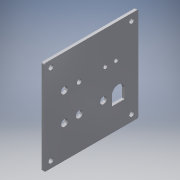
# Autodesk Inventor part: PP-LAS-0001
Saved by Autodesk Inventor 2018.3 (Build 223284000, 284)
## iProperties
Created: 2021-05-05
Part Number: PP-LAS-0001
Material: Plástico ABS
Document SubType Name: Modeling
Designer: L.Aguerre
Density: 1.06 g/cm^3
Appearance: Suave - Blanco
Description: FRENTE DE PANEL SERIGRAFIADO
Author: laguerre
Autodesk Inventor part; units mm, degrees
ref_plane "YZ Plane" through (0, 0, 0) normal (1, 0, 0) x (0, 1, 0)
ref_plane "XZ Plane" through (0, 0, 0) normal (0, 1, 0) x (-1, 0, 0)
ref_plane "XY Plane" through (0, 0, 0) normal (0, 0, 1) x (1, 0, 0)
sketch "Boceto39" plane through (0, 0, 0) normal (0, 0, 1) x (1, 0, 0)
  line L0 (-34, 35) -> (34, 35)
  line L1 (35, 34) -> (35, -34)
  line L2 (34, -35) -> (-34, -35)
  line L3 (-35, -34) -> (-35, 34)
  arc A0 (-34, 35) -> (-35, 34) centre (-34, 34) ccw
  arc A1 (35, 34) -> (34, 35) centre (34, 34) ccw
  arc A2 (34, -35) -> (35, -34) centre (34, -34) ccw
  arc A3 (-35, -34) -> (-34, -35) centre (-34, -34) ccw
  point P0 (0, 0)
  point P1 (0, 35)
  point P2 (-35, 0)
  dimension "d373" = 70
  dimension "d374" = 70
  dimension "d375" = 1
  constraints: 8 end point, 8 point on circle, 8 tangent, 4 centre point, 3 equal radius, 2 midpoint, 2 parallel, 1 horizontal, 1 horizontal alignment, 1 perpendicular, 1 vertical alignment
  measures "d373" distance between parallel lines of L1 L3
  measures "d374" distance between parallel lines of L2 L0
  measures "d375" radius of A0
extrude "Extrusión13" add sketch "Boceto39" along normal blind 2
sketch "Boceto43" plane through (0, 0, 2) normal (0, 0, 1) x (1, 0, 0)
  line L0 (-30, 30) -> (30, 30) construction
  line L1 (30, 30) -> (30, -30) construction
  line L2 (30, -30) -> (-30, -30) construction
  line L3 (-30, -30) -> (-30, 30) construction
  point P0 (0, 0)
  point P1 (0, 30)
  point P2 (-30, 0)
  dimension "d402" = 60
  constraints: 8 end point, 2 coincident, 2 midpoint, 2 parallel, 2 perpendicular, 1 horizontal, 1 horizontal alignment, 1 point on line, 1 vertical alignment
  measures "d402" distance of L0.start L0.end
hole "Agujero2" at (30, 30, 2) at (30, -30, 2) at (-30, -30, 2) at (-30, 30, 2) direction (0, 0, -1) diameter 3.5 depth 8 tip angle 118
sketch "Boceto40" plane through (0, 0, 2) normal (0, 0, 1) x (1, 0, 0)
  line L0 (-25, 0) -> (-4, 0)
  line L1 (-2, -2) -> (-2, -18)
  line L2 (-4, -20) -> (-25, -20)
  line L3 (-27, -18) -> (-27, -2)
  line L4 (4, 0) -> (25, 0)
  line L5 (27, -2) -> (27, -18)
  line L6 (25, -20) -> (4, -20)
  line L7 (2, -18) -> (2, -2)
  line L8 (-25, 20) -> (25, 20)
  line L9 (27, 18) -> (27, 5)
  line L10 (25, 3) -> (-25, 3)
  line L11 (-27, 5) -> (-27, 18)
  arc A0 (-27, -18) -> (-25, -20) centre (-25, -18) ccw
  arc A1 (-4, -20) -> (-2, -18) centre (-4, -18) ccw
  arc A2 (-2, -2) -> (-4, 0) centre (-4, -2) ccw
  arc A3 (-25, 0) -> (-27, -2) centre (-25, -2) ccw
  arc A4 (4, 0) -> (2, -2) centre (4, -2) ccw
  arc A5 (2, -18) -> (4, -20) centre (4, -18) ccw
  arc A6 (25, -20) -> (27, -18) centre (25, -18) ccw
  arc A7 (27, -2) -> (25, 0) centre (25, -2) ccw
  line L12 (-34, -35) -> (34, -35) projected
  arc A8 (-27, 5) -> (-25, 3) centre (-25, 5) ccw
  arc A9 (-25, 20) -> (-27, 18) centre (-25, 18) ccw
  arc A10 (27, 18) -> (25, 20) centre (25, 18) ccw
  arc A11 (25, 3) -> (27, 5) centre (25, 5) ccw
  line L13 (25, 19.7) -> (-25, 19.7)
  arc A12 (-25, 19.7) -> (-26.7, 18) centre (-25, 18) ccw
  line L14 (-26.7, 18) -> (-26.7, 5)
  arc A13 (-26.7, 5) -> (-25, 3.3) centre (-25, 5) ccw
  line L15 (-25, 3.3) -> (25, 3.3)
  arc A14 (25, 3.3) -> (26.7, 5) centre (25, 5) ccw
  line L16 (26.7, 5) -> (26.7, 18)
  arc A15 (26.7, 18) -> (25, 19.7) centre (25, 18) ccw
  line L17 (-4, -0.3) -> (-25, -0.3)
  arc A16 (-25, -0.3) -> (-26.7, -2) centre (-25, -2) ccw
  line L18 (-26.7, -2) -> (-26.7, -18)
  arc A17 (-26.7, -18) -> (-25, -19.7) centre (-25, -18) ccw
  line L19 (-25, -19.7) -> (-4, -19.7)
  arc A18 (-4, -19.7) -> (-2.3, -18) centre (-4, -18) ccw
  line L20 (-2.3, -18) -> (-2.3, -2)
  arc A19 (-2.3, -2) -> (-4, -0.3) centre (-4, -2) ccw
  line L21 (25, -0.3) -> (4, -0.3)
  arc A20 (4, -0.3) -> (2.3, -2) centre (4, -2) ccw
  line L22 (2.3, -2) -> (2.3, -18)
  arc A21 (2.3, -18) -> (4, -19.7) centre (4, -18) ccw
  line L23 (4, -19.7) -> (25, -19.7)
  arc A22 (25, -19.7) -> (26.7, -18) centre (25, -18) ccw
  line L24 (26.7, -18) -> (26.7, -2)
  arc A23 (26.7, -2) -> (25, -0.3) centre (25, -2) ccw
  point P0 (0, 0)
  point P1 (-27, 0)
  point P2 (-2, -20)
  point P3 (-27, -20)
  point P4 (27, -20)
  point P5 (2, -20)
  point P6 (0, 20)
  dimension "d378" = 2
  dimension "d379" = 2
  dimension "d380" = 25
  dimension "d381" = 25
  dimension "d382" = 20
  dimension "d383" = 2
  dimension "d385" = 3
  dimension "d386" = 2
  dimension "d387" = 17
  dimension "d388" = 0.3
  dimension "d389" = 0.3
  dimension "d390" = 0.3
  dimension "d477" = 20
  constraints: 48 end point, 48 point on circle, 24 centre point, 24 tangent, 12 parallel, 10 equal radius, 10 point on line, 6 perpendicular, 3 collinear, 3 horizontal, 1 midpoint, 1 vertical alignment, 21 other
  measures "d378" distance from line of point (0, 0) L1
  measures "d379" distance from line of point (0, 0) L7
  measures "d380" distance of point (-2, -20) point (-27, -20)
  measures "d381" distance of point (27, -20) point (2, -20)
  measures "d382" distance of point (-27, -20) point (-27, 0)
  measures "d383" radius of A0
  measures "d385" distance between parallel lines of L10 L0
  measures "d386" radius of A8
  measures "d387" distance between parallel lines of L8 L10
  measures "d388" distance between parallel lines of L15 L10
  measures "d389" distance between parallel lines of L4 L21
  measures "d390" distance between parallel lines of L0 L17
  measures "d477" distance from line of L6 point (0, 0)
extrude "Extrusión14" add sketch "Boceto40" along normal blind 0.001
sketch "Boceto41" plane through (0, 0, 2) normal (0, 0, 1) x (1, 0, 0)
  circle A0 centre (-20, -10.7) radius 5 construction
  line L0 (-34, -35) -> (34, -35) projected
  line L1 (-35, 34) -> (-35, -34) projected
  circle A1 centre (-9, -10.7) radius 2.5
  line L2 (-20, -10.7) -> (-9, -10.7) construction
  line L3 (-4, -19.7) -> (-25, -19.7) projected
  circle A2 centre (9, -10.7) radius 2.5
  circle A3 centre (20, -10.7) radius 2.5
  line L4 (25, -19.7) -> (4, -19.7) projected
  circle A4 centre (-18.5, 10.3) radius 1.5
  circle A5 centre (-10.5, 10.3) radius 1.5
  line L5 (-18.5, 10.3) -> (-10.5, 10.3) construction
  line L6 (25, 3.3) -> (-25, 3.3) projected
  circle A6 centre (20, 10.3) radius 2.5
  circle A7 centre (9, 10.3) radius 1.75
  line L7 (9, -10.7) -> (20, -10.7) construction
  line L8 (9, 10.3) -> (20, 10.3) construction
  line L9 (-24.7, -10.7) -> (-24.7, -17.7)
  line L10 (-24.7, -17.7) -> (-15.3, -17.7)
  line L11 (-15.3, -17.7) -> (-15.3, -10.7)
  arc A8 (-15.3, -10.7) -> (-24.7, -10.7) centre (-20, -10.7) ccw
  line L12 (-20, -6) -> (-22.9713, -6) construction
  point P0 (0, 0)
  point P1 (-14.5, -10.7)
  point P2 (-14.5, -19.7)
  point P3 (-14.5, 10.3)
  point P4 (14.5, -10.7)
  point P5 (14.5, -19.7)
  point P6 (14.5, 10.3)
  point P7 (-20, -17.7)
  dimension "d393" = 10
  dimension "d396" = 5
  dimension "d397" = 11
  dimension "d399" = 11
  dimension "d410" = 9
  dimension "d415" = 3
  dimension "d416" = 7
  dimension "d417" = 8
  dimension "d418" = 3.5
  dimension "d419" = 11
  dimension "d474" = 9.4
  dimension "d475" = 7
  dimension "d476" = 4.7
  constraints: 16 end point, 9 centre point, 7 midpoint, 5 horizontal, 5 horizontal alignment, 5 vertical alignment, 4 equal radius, 3 point on circle, 3 tangent, 2 perpendicular, 1 coincident, 1 vertical
  measures "d393" diameter of A0
  measures "d396" diameter of A1
  measures "d397" distance of L2.start L2.end
  measures "d399" distance of L7.end L7.start
  measures "d410" distance between parallel lines of L2 L3
  measures "d415" diameter of A5
  measures "d416" distance between parallel lines of L5 L6
  measures "d417" distance of L5.start L5.end
  measures "d418" diameter of A7
  measures "d419" distance of L8.end L8.start
  measures "d474" distance of L9.end L10.end
  measures "d475" distance from line of L2.start L10
  measures "d476" distance from line of L2.start L12
extrude "Extrusión15" cut sketch "Boceto41" against normal blind 2
sketch "Boceto42" plane through (0, 0, 2) normal (0, 0, 1) x (1, 0, 0)
  line L0 (-19.9009, -2.7) -> (-1.3327, -2.7) construction
  line L1 (-1.3327, -2.7) -> (-1.3327, -6.6561) construction
  line L2 (-1.3327, -6.6561) -> (-19.9009, -6.6561) construction
  line L3 (-19.9009, -6.6561) -> (-19.9009, -2.7) construction
  line L4 (-11.8025, -15.7) -> (-8.1255, -15.7) construction
  line L5 (-8.1255, -15.7) -> (-8.1255, -16.9024) construction
  line L6 (-8.1255, -16.9024) -> (-11.8025, -16.9024) construction
  line L7 (-11.8025, -16.9024) -> (-11.8025, -15.7) construction
  line L8 (6.4191, -2.7) -> (25.511, -2.7) construction
  line L9 (25.511, -2.7) -> (25.511, -5.9558) construction
  line L10 (25.511, -5.9558) -> (6.4191, -5.9558) construction
  line L11 (6.4191, -5.9558) -> (6.4191, -2.7) construction
  line L12 (7.0108, -15.7) -> (12.5482, -15.7) construction
  line L13 (12.5482, -15.7) -> (12.5482, -16.8686) construction
  line L14 (12.5482, -16.8686) -> (7.0108, -16.8686) construction
  line L15 (7.0108, -16.8686) -> (7.0108, -15.7) construction
  line L16 (17.6981, -15.7) -> (23.2355, -15.7) construction
  line L17 (23.2355, -15.7) -> (23.2355, -15.9466) construction
  line L18 (23.2355, -15.9466) -> (17.6981, -15.9466) construction
  line L19 (17.6981, -15.9466) -> (17.6981, -15.7) construction
  circle A0 centre (9, -10.7) radius 2.5 projected
  line L20 (-18.1999, 5.1784) -> (-18.1999, 6.3) construction
  line L21 (-18.1999, 6.3) -> (-6.5736, 6.3) construction
  line L22 (-6.5736, 6.3) -> (-6.5736, 5.1784) construction
  line L23 (-6.5736, 5.1784) -> (-18.1999, 5.1784) construction
  line L24 (6.4525, 5.7678) -> (6.4525, 6.3) construction
  line L25 (6.4525, 6.3) -> (10.1295, 6.3) construction
  line L26 (10.1295, 6.3) -> (10.1295, 5.7678) construction
  line L27 (10.1295, 5.7678) -> (6.4525, 5.7678) construction
  circle A1 centre (-18.5, 10.3) radius 1.5 projected
  line L28 (-22.5122, 16.6992) -> (-6.3487, 16.6992) construction
  line L29 (-6.3487, 16.6992) -> (-6.3487, 14.435) construction
  line L30 (-6.3487, 14.435) -> (-22.5122, 14.435) construction
  line L31 (-22.5122, 14.435) -> (-22.5122, 16.6992) construction
  line L32 (6.7652, 14.2645) -> (6.7652, 16.6992) construction
  line L33 (6.7652, 16.6992) -> (24.191, 16.6992) construction
  line L34 (24.191, 16.6992) -> (24.191, 14.2645) construction
  line L35 (24.191, 14.2645) -> (6.7652, 14.2645) construction
  line L36 (17.5924, 5.1479) -> (17.5924, 6.3) construction
  line L37 (17.5924, 6.3) -> (21.2695, 6.3) construction
  line L38 (21.2695, 6.3) -> (21.2695, 5.1479) construction
  line L39 (21.2695, 5.1479) -> (17.5924, 5.1479) construction
  point P0 (0, 0)
  dimension "d411" = 5
  dimension "d412" = 8
  dimension "d420" = 4
  constraints: 6 collinear, 20 other
  measures "d411" distance from line of A0.centre L12
  measures "d412" distance from line of L8 A0.centre
  measures "d420" distance from line of A1.centre L21
sketch "Boceto44" plane through (0, 0, 2) normal (0, 0, 1) x (1, 0, 0)
  line L0 (34, 35) -> (-34, 35) projected
  line L1 (25, 20) -> (-25, 20) projected
  line L2 (-2.9167, 30) -> (2.9167, 30) construction
  line L3 (2.9167, 30) -> (2.9167, 24) construction
  line L4 (2.9167, 24) -> (-2.9167, 24) construction
  line L5 (-2.9167, 24) -> (-2.9167, 30) construction
  line L6 (-2.9167, 26.5) -> (-1.6167, 26.5)
  line L7 (-1.6167, 26.5) -> (-1.6167, 25.5)
  line L8 (-1.6167, 25.5) -> (-2.9167, 25.5)
  line L9 (-2.9167, 25.5) -> (-2.9167, 26.5)
  line L10 (-1.5167, 25.5) -> (-0.5167, 25.5)
  line L11 (-0.5167, 25.5) -> (-0.5167, 24)
  line L12 (-0.5167, 24) -> (-1.5167, 24)
  line L13 (-1.5167, 24) -> (-1.5167, 25.5)
  line L14 (-0.4167, 25.5) -> (1.6833, 25.5)
  line L15 (1.6833, 25.5) -> (2.9167, 26.7333)
  line L16 (2.9167, 26.7333) -> (2.9167, 28.7667)
  line L17 (2.9167, 28.7667) -> (1.6833, 30)
  line L18 (1.6833, 30) -> (-0.2833, 30)
  line L19 (-1.5167, 28.7667) -> (-0.2833, 30)
  line L20 (-1.5167, 28.7667) -> (-1.5167, 26.5)
  line L21 (-0.5167, 26.5) -> (-1.5167, 26.5)
  line L22 (-0.4167, 26.5) -> (1.2691, 26.5)
  line L23 (1.2691, 26.5) -> (1.9167, 27.1475)
  line L24 (1.9167, 27.1475) -> (1.9167, 28.3525)
  line L25 (1.9167, 28.3525) -> (1.2691, 29)
  line L26 (1.2691, 29) -> (0.1309, 29)
  line L27 (0.1309, 29) -> (-0.5167, 28.3525)
  line L28 (-0.5167, 28.3525) -> (-0.5167, 26.5)
  line L29 (-0.4167, 26.5) -> (-0.4167, 25.5)
  point P0 (0, 0)
  point P1 (0, 35)
  point P2 (0, 35)
  point P3 (0, 30)
  dimension "d449" = 5
  dimension "d450" = 6
  dimension "d451" = 1
  dimension "d452" = 3.5
  dimension "d453" = 1.3
  dimension "d454" = 1
  dimension "d455" = 0.1
  dimension "d457" = 45
  dimension "d461" = 0.1
  dimension "d463" = 1
  dimension "d464" = 1
  dimension "d465" = 1
  dimension "d466" = 1
  dimension "d467" = 1
  dimension "d468" = 4.6
  constraints: 48 end point, 8 perpendicular, 7 parallel, 6 collinear, 6 point on line, 4 horizontal, 3 midpoint, 3 vertical, 1 vertical alignment, 2 other
  measures "d449" distance between parallel lines of L0 L2
  measures "d450" distance of L2.end L3.end
  measures "d451" distance between parallel lines of L8 L6
  measures "d452" distance between parallel lines of L2 L6
  measures "d453" distance of L7.end L8.end
  measures "d454" distance between parallel lines of L13 L11
  measures "d455" distance between parallel lines of L7 L13
  measures "d457" angle of L23 L22
  measures "d461" distance between parallel lines of L29 L11
  measures "d463" distance between parallel lines of L15 L23
  measures "d464" distance between parallel lines of L19 L27
  measures "d465" distance between parallel lines of L2 L26
  measures "d466" distance between parallel lines of L16 L24
  measures "d467" distance between parallel lines of L17 L25
  measures "d468" distance from line of L5 L14.end
sketch "Boceto45" plane through (0, 0, 2) normal (0, 0, 1) x (1, 0, 0)
  line L0 (-14.5048, -25.2952) -> (14.5048, -25.2952) construction
  line L1 (14.5048, -25.2952) -> (14.5048, -27.5438) construction
  line L2 (14.5048, -27.5438) -> (-14.5048, -27.5438) construction
  line L3 (-14.5048, -27.5438) -> (-14.5048, -25.2952) construction
  line L4 (-34, -35) -> (34, -35) projected
  point P0 (0, 0)
  point P1 (0, -25.2952)
  constraints: 1 midpoint, 1 vertical alignment, 2 other
